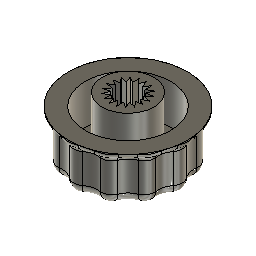
volume_knob (Autodesk Fusion 360 design; units mm, degrees)
Autodesk Fusion 360 part; units mm, degrees
sketch "Skizze1" plane through (0, 0, 0) normal (0, 0, 1) x (1, 0, 0)
  arc A0 (3.951698, -9.338845) -> (2.523801, -9.418955) centre (3.429668, -12.799695) ccw
  circle A1 centre (0, 0) radius 5
  line L0 (-1.356886, -7.695284) -> (1.126342, 6.387801) construction
  line L1 (5.775232, 21.553458) -> (-3.705632, -13.829606) construction
  arc A2 (6.895153, -6.895153) -> (6.111828, -8.091692) centre (9.370027, -9.370027) ccw
  line L2 (2.4, -0.000006) -> (3.545308, -0.625133)
  arc A3 (-1.247152, -10.063526) -> (1.247152, -10.063525) centre (0, -8.5) ccw
  arc A4 (-9.418955, -2.523801) -> (-10.063525, -1.247152) centre (-12.799695, -3.429668) ccw
  line L3 (2.25526, -0.820854) -> (3.117691, -1.8)
  line L4 (-0.416762, -2.363537) -> (-1.231273, -3.382893)
  line L5 (-5.895645, 22.002848) -> (3.63479, -13.565219) construction
  line L6 (3.117691, -1.8) -> (1.838507, -1.54269)
  arc A5 (10.063526, -1.247152) -> (10.063525, 1.247152) centre (8.5, 0) ccw
  circle A6 centre (0, 0) radius 2.4 construction
  circle A7 centre (0, 0) radius 11.5
  circle A8 centre (0, 0) radius 10.5 construction
  line L7 (0, -60.68219) -> (0, 59.394716) construction
  circle A9 centre (0, 0) radius 8.25
  line L8 (-3.545308, -0.625133) -> (-2.4, 0)
  line L9 (-1.83851, -1.542686) -> (-3.117691, -1.8)
  circle A10 centre (0, 0) radius 3.6 construction
  line L10 (-2.255264, -0.820843) -> (-3.545308, -0.625133)
  arc A11 (-10.063526, 1.247152) -> (-10.063525, -1.247152) centre (-8.5, 0) ccw
  arc A12 (3.951698, -9.338845) -> (6.111828, -8.091692) centre (4.25, -7.361216) ccw
  line L11 (-1.165017, 6.60714) -> (1.472183, -8.349163) construction
  arc A13 (-2.523801, -9.418955) -> (-3.951697, -9.338845) centre (-3.429668, -12.799695) ccw
  line L12 (3.545308, -0.625133) -> (2.255262, -0.820848)
  line L13 (1.838503, -1.542695) -> (2.314035, -2.75776)
  line L14 (0, -3.6) -> (-0.416756, -2.363539)
  line L15 (0.41675, -2.36354) -> (0, -3.6)
  arc A14 (-6.111828, -8.091693) -> (-3.951697, -9.338845) centre (-4.25, -7.361216) ccw
  arc A15 (-9.338845, -3.951698) -> (-8.091692, -6.111828) centre (-7.361216, -4.25) ccw
  line L16 (-1.231273, -3.382893) -> (-1.2, -2.078461)
  line L17 (-3.117691, -1.8) -> (-2.255262, -0.820848)
  arc A16 (2.523801, -9.418955) -> (1.247152, -10.063525) centre (3.429668, -12.799695) ccw
  line L18 (2.314035, -2.75776) -> (1.2, -2.078461)
  arc A17 (8.091693, -6.111828) -> (9.338845, -3.951697) centre (7.361216, -4.25) ccw
  arc A18 (-9.338845, -3.951698) -> (-9.418955, -2.523801) centre (-12.799695, -3.429668) ccw
  line L19 (-1.200005, -2.078458) -> (-2.314035, -2.75776)
  arc A19 (-8.091693, 6.111828) -> (-9.338845, 3.951697) centre (-7.361216, 4.25) ccw
  line L20 (-2.314035, -2.75776) -> (-1.838507, -1.54269)
  arc A20 (9.338845, 3.951698) -> (8.091692, 6.111828) centre (7.361216, 4.25) ccw
  arc A21 (-1.247152, -10.063526) -> (-2.523801, -9.418955) centre (-3.429668, -12.799695) ccw
  arc A22 (-10.063526, 1.247152) -> (-9.418955, 2.523801) centre (-12.799695, 3.429668) ccw
  arc A23 (-6.895153, -6.895153) -> (-8.091692, -6.111828) centre (-9.370027, -9.370027) ccw
  line L21 (-0.41675, 2.36354) -> (0, 3.6)
  circle A24 centre (0, 8.5) radius 2 construction
  arc A25 (10.063526, -1.247152) -> (9.418955, -2.523801) centre (12.799695, -3.429668) ccw
  line L22 (-1.838503, 1.542695) -> (-2.314035, 2.75776)
  arc A26 (-8.091693, 6.111828) -> (-6.895153, 6.895153) centre (-9.370027, 9.370027) ccw
  arc A27 (8.091693, -6.111828) -> (6.895153, -6.895153) centre (9.370027, -9.370027) ccw
  arc A28 (-6.895153, 6.895153) -> (-6.111828, 8.091692) centre (-9.370027, 9.370027) ccw
  line L23 (1.231273, -3.382893) -> (0.416756, -2.363539)
  arc A29 (1.247152, 10.063526) -> (2.523801, 9.418955) centre (3.429668, 12.799695) ccw
  arc A30 (9.418955, 2.523801) -> (10.063525, 1.247152) centre (12.799695, 3.429668) ccw
  arc A31 (-6.111828, -8.091693) -> (-6.895153, -6.895153) centre (-9.370027, -9.370027) ccw
  line L24 (-1.231273, 3.382893) -> (-0.416756, 2.363539)
  arc A32 (6.111828, 8.091693) -> (3.951697, 9.338845) centre (4.25, 7.361216) ccw
  arc A33 (9.418955, -2.523801) -> (9.338845, -3.951697) centre (12.799695, -3.429668) ccw
  circle A34 centre (3.429668, 12.799695) radius 3.5 construction
  line L25 (1.199995, -2.078464) -> (1.231273, -3.382893)
  arc A35 (-3.951698, 9.338845) -> (-2.523801, 9.418955) centre (-3.429668, 12.799695) ccw
  arc A36 (1.247152, 10.063526) -> (-1.247152, 10.063525) centre (0, 8.5) ccw
  line L26 (2.255264, 0.820843) -> (3.545308, 0.625133)
  line L27 (-2.314035, 2.75776) -> (-1.2, 2.078461)
  circle A37 centre (-3.429668, 12.799695) radius 3.5 construction
  arc A38 (6.895153, 6.895153) -> (8.091692, 6.111828) centre (9.370027, 9.370027) ccw
  arc A39 (2.523801, 9.418955) -> (3.951697, 9.338845) centre (3.429668, 12.799695) ccw
  arc A40 (6.111828, 8.091693) -> (6.895153, 6.895153) centre (9.370027, 9.370027) ccw
  line L28 (-2.25526, 0.820854) -> (-3.117691, 1.8)
  arc A41 (-9.418955, 2.523801) -> (-9.338845, 3.951697) centre (-12.799695, 3.429668) ccw
  arc A42 (-2.523801, 9.418955) -> (-1.247152, 10.063525) centre (-3.429668, 12.799695) ccw
  arc A43 (-3.951698, 9.338845) -> (-6.111828, 8.091692) centre (-4.25, 7.361216) ccw
  line L29 (1.200005, 2.078458) -> (2.314035, 2.75776)
  arc A44 (9.338845, 3.951698) -> (9.418955, 2.523801) centre (12.799695, 3.429668) ccw
  line L30 (0.416762, 2.363537) -> (1.231273, 3.382893)
  line L31 (2.314035, 2.75776) -> (1.838507, 1.54269)
  line L32 (1.231273, 3.382893) -> (1.2, 2.078461)
  line L33 (3.117691, 1.8) -> (2.255262, 0.820848)
  line L34 (0, 3.6) -> (0.416756, 2.363539)
  line L35 (-2.4, 0.000006) -> (-3.545308, 0.625133)
  line L36 (1.83851, 1.542686) -> (3.117691, 1.8)
  line L37 (-3.545308, 0.625133) -> (-2.255262, 0.820848)
  line L38 (-1.199995, 2.078464) -> (-1.231273, 3.382893)
  line L39 (-3.117691, 1.8) -> (-1.838507, 1.54269)
  line L40 (3.545308, 0.625133) -> (2.4, 0)
  line L41 (-196.099114, 0) -> (114.973446, 0) construction
  point P0 (-1.247152, 10.063525)
  point P1 (1.247152, 10.063526)
  dimension "d2" = 360
  dimension "d4" = 360
  dimension "d5" = 7.2
  dimension "d6" = 1.2
  dimension "d7" = 10
  dimension "d8" = 10
  dimension "d9" = 10
  dimension "d10" = 16.5
  dimension "d11" = 21
  dimension "d12" = 23
  dimension "d13" = 4
  dimension "d14" = 15
  dimension "d15" = 7
  dimension "d16" = 15
  dimension "d17" = 7
  constraint horizontal L41
  constraint vertical L7
  constraint coincident A1.centre L41
  constraint coincident A1.centre L7
  constraint concentric A6 A10
  constraint coincident A1.centre L11
  constraint coincident A1.centre L0
  constraint coincident L21.end A10
  constraint coincident L21.end L7
  constraint concentric A1 A10
  constraint concentric A9 A10
  constraint concentric A1 A8
  constraint concentric A6 A7
  constraint coincident A24.centre L7
  constraint tangent A8 A24
  constraint coincident A1.centre L1
  constraint tangent A24 A34
  constraint coincident A1.centre L5
  constraint tangent A24 A37
  constraint coincident A24.centre A36.centre
  measures "d5" diameter of A10
  measures "d6" distance of A6 A10
  measures "d7" angle of L7 L11
  measures "d8" angle of L0 L7
  measures "d9" diameter of A1
  measures "d10" diameter of A9
  measures "d11" diameter of A8
  measures "d12" diameter of A7
  measures "d13" diameter of A24
  measures "d14" angle of L1 L7
  measures "d15" diameter of A34
  measures "d16" angle of L5 L7
  measures "d17" diameter of A37
extrude "Extrusion1" add sketch "Skizze1" along normal blind 10 contours A1 picked at (-2.015103, -3.49026)
extrude "Extrusion2" add sketch "Skizze1" against normal blind 2 contours A0 A2 A3 A4 A5 A11 A12 A13 A14 A15 A16 A17 A18 A19 A20 A21 A22 A23 A25 A26 A27 A28 A29 A30 A31 A32 A33 A35 A36 A38 A39 A40 A41 A42 A43 A44 | A1 | L2 L3 L4 L6 L8 L9 L10 L12 L13 L14 L15 L16 L17 L18 L19 L20 L21 L22 L23 L24 L25 L26 L27 L28 L29 L30 L31 L32 L33 L34 L35 L36 L37 L38 L39 L40 | A9 picked at (-7.804209, -4.448226) picked at (-2.015103, -3.49026) picked at (-0.612834, 0.514232) picked at (7.135951, -0.409866)
extrude "Extrusion3" add sketch "Skizze1" along normal blind 7.7 contours A0 A2 A3 A4 A5 A11 A12 A13 A14 A15 A16 A17 A18 A19 A20 A21 A22 A23 A25 A26 A27 A28 A29 A30 A31 A32 A33 A35 A36 A38 A39 A40 A41 A42 A43 A44 | A7 picked at (-7.804209, -4.448226) picked at (10.645073, 2.391233)
extrude "Extrusion4" cut sketch "Skizze1" along normal blind 6.7 contours A7 picked at (10.645073, 2.391233)
fillet "Abrundung1" radius 1 1 faces at (10.645073, 2.391233, 6.7)
fillet "Abrundung2" radius 2 1 faces at (-0.61585, 2.298384, -2)
